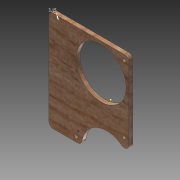
# Autodesk Inventor part: p1
Saved by Autodesk Inventor 2015 (Build 190159000, 159)
## iProperties
Created: 2016-02-03
Part Number: p1
Material: Generic
Document SubType Name: Modeling
Designer: david
Density: 1 g/cm^3
Appearance: Birch - Natural Polished
Author: david
Autodesk Inventor part; units mm, degrees
ref_plane "YZ Plane" through (0, 0, 0) normal (1, 0, 0) x (0, 1, 0)
ref_plane "XZ Plane" through (0, 0, 0) normal (0, 1, 0) x (-1, 0, 0)
ref_plane "XY Plane" through (0, 0, 0) normal (0, 0, 1) x (1, 0, 0)
sketch "Sketch1" plane through (0, 0, 0) normal (0, 1, 0) x (-1, 0, 0)
  line L0 (20, 45) -> (-20, 45)
  line L1 (-20, 45) -> (-20, -45)
  line L2 (-20, -45) -> (20, -45)
  line L3 (20, -45) -> (20, 45)
  line L4 (20, 45) -> (-20, -45) construction
  line L5 (-20, 45) -> (20, -45) construction
  arc A0 (-20, -45) -> (20, -45) centre (0, -45) ccw
  line L6 (20, -45) -> (52, -45)
  line L7 (52, -45) -> (52, 45)
  line L8 (52, 45) -> (20, 45)
  line L9 (20, 45) -> (20, -45)
  point P0 (0, 0)
  dimension "d0" = 40
  dimension "d1" = 90
  dimension "d7" = 32
  dimension "d8" = 90
  constraints: 20 end point, 4 parallel, 3 midpoint, 2 horizontal, 2 perpendicular, 2 point on circle, 1 centre point
  measures "d0" distance of L2.end L1.end
  measures "d1" distance of L1.end L0.end
  measures "d7" distance of L8.end L7.end
  measures "d8" distance of L7.end L6.end
extrude "Extrusion1" add sketch "Sketch1" along normal blind 3.6
sketch "Sketch3" plane through (0, 3.6, 0) normal (0, 1, 0) x (1, 0, 0)
  arc A0 (20, 45) -> (-20, 45) centre (0, 45) ccw projected
  circle A1 centre (0, 45) radius 20
  circle A2 centre (0, 45) radius 22.5
  point P0 (0, 0)
  point P1 (-19.7203, 38.3333)
  dimension "d13" = 45
  constraints: 2 coincident, 1 centre point, 1 horizontal alignment, 3 other
  measures "d13" diameter of A2
extrude "Extrusion3" cut sketch "Sketch3" against normal blind 10 contours A1 A0 | A2
fillet "Fillet2" radius 4 5 edges at (-52, 1.8, -45) (-52, 1.8, 45) (20, 1.8, 45) (-22.5, 1.8, -45) (20, 1.8, -34.6922)
sketch "Sketch4" plane through (0, 3.6, 0) normal (0, 1, 0) x (1, 0, 0)
  circle A0 centre (-5, -20) radius 22.5
  line L0 (20, -41) -> (20, 23.8754) projected
  line L1 (-48, -45) -> (16, -45) projected
  point P0 (0, 0)
  dimension "d14" = 45
  dimension "d15" = 25
  dimension "d16" = 25
  constraints: 1 centre point
  measures "d14" diameter of A0
  measures "d15" distance from line of L0 A0.centre
  measures "d16" distance from line of L1 A0.centre
extrude "Extrusion4" cut sketch "Sketch4" against normal blind 10
sketch "Sketch5" plane through (0, 0, 0) normal (0, -1, 0) x (1, 0, 0)
  circle A0 centre (-27.5, -40.5) radius 1.625
  circle A1 centre (15.5, 40.5) radius 1.625
  circle A2 centre (15.5, -19.5) radius 1.625
  line L0 (20, 41) -> (20, -23.8754) projected
  line L1 (-48, 45) -> (16, 45) projected
  line L2 (-26.1964, -45) -> (-48, -45) projected
  line L3 (-52, -41) -> (-52, 41) projected
  point P0 (0, 0)
  dimension "d19" = 3.25
  dimension "d21" = 3.25
  dimension "d22" = 3.25
  dimension "d23" = 4.5
  dimension "d24" = 4.5
  dimension "d25" = 4.5
  dimension "d26" = 56.75
  dimension "d27" = 4.5
  dimension "d28" = 24.5
  constraints: 3 centre point
  measures "d19" diameter of A0
  measures "d21" diameter of A1
  measures "d22" diameter of A2
  measures "d23" distance from line of L0 A2.centre
  measures "d24" distance from line of L0 A1.centre
  measures "d25" distance from line of L1 A1.centre
  measures "d27" distance from line of L2 A0.centre
  measures "d28" distance from line of L3 A0.centre
extrude "Extrusion5" cut sketch "Sketch5" against normal blind 10
sketch "Sketch6" plane through (0, 3.6, 0) normal (0, 1, 0) x (1, 0, 0)
  circle A0 centre (-48, -40) radius 1.575
  line L0 (-48, -45) -> (16, -45) projected
  line L1 (-52, 41) -> (-52, -41) projected
  point P0 (0, 0)
  dimension "d31" = 3.15
  dimension "d32" = 5
  dimension "d33" = 4
  constraints: 1 centre point
  measures "d31" diameter of A0
  measures "d32" distance from line of L0 A0.centre
  measures "d33" distance from line of L1 A0.centre
extrude "Extrusion6" cut sketch "Sketch6" against normal blind 10
body "Solid1"
